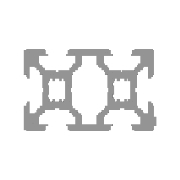
# Autodesk Inventor part: 2040Vslot
Saved by Autodesk Inventor 2023 (Build 270158000, 158)
## iProperties
IsCustomPart: 1
Created: 2023-08-15
Part Number: 2040Vslot
Material: Aluminum 6061
Description: STEP AP214
Document SubType Name: Modeling
Designer: Felix
Language: en-US
Size Designation: (Unnamed 1)
Categories: <MemberInstance><Categories><Category DisplayName="Structural Shapes" InternalName="089c4875-fa83-4c05-b084-43b9cc11f5ed" Mnemonic="GRDR"><CategoryParameter DisplayName="Mass per Length Unit" InternalName="0bb95a10-148f-4027-a459-38d7b056702a" Mnemonic="shpmass"/><CategoryParameter DisplayName="Section Area" InternalName="1ff91680-64b0-4202-b9a3-7fd3f94bba3b" Mnemonic="secarea"/><CategoryParameter DisplayName="Radius of Gyration (x)" InternalName="25778675-03e9-40c1-b6a8-4a9ed693320d" Mnemonic="gyrradx"/><CategoryParameter DisplayName="Torsional Rigidity Modulus" InternalName="26c1ec35-5026-4c63-ad0a-751cf684a536" Mnemonic="torrigmod"/><CategoryParameter DisplayName="Distance of the Center of Gravity X-X" InternalName="26c9bdb8-9c79-4b4f-a92e-8e197583c9c4" Mnemonic="grcendistX"/><CategoryParameter DisplayName="Legacy Member ID" InternalName="340afe4f-75d7-48d3-ab7d-943f3c3da468" Mnemonic="LegacyMemberID"/><CategoryParameter DisplayName="Base Length" InternalName="42e34263-8f20-4d0e-ad48-bf1385b87c24" Mnemonic="shplen"/><CategoryParameter DisplayName="Moment of Inertia (y)" InternalName="4b9f58ea-bced-460e-81ea-3d29ca5a49e3" Mnemonic="inermomy"/><CategoryParameter DisplayName="Moment of Inertia (x)" InternalName="4cd780bc-73d7-43ac-917a-579e5cbd684d" Mnemonic="inermomx"/><CategoryParameter DisplayName="Custom Base Point" InternalName="4f1d1b73-316d-484b-a3df-9cbabb16eb77" Mnemonic="shpBasePoint"/><CategoryParameter DisplayName="Shape Height" InternalName="50274e7d-5ac0-4796-92cb-c59e54983c67" Mnemonic="shpheig"/><CategoryParameter DisplayName="Section Module (y)" InternalName="59eaa5e9-d227-48dc-b6c1-6920f96e0f95" Mnemonic="secmody"/><CategoryParameter DisplayName="Section Designation" InternalName="5a64d034-428d-49c8-ba32-7619764de20f" Mnemonic="shpdes"/><CategoryParameter DisplayName="Section Module (x)" InternalName="72cfad18-cf51-4ed4-aaa7-c6b224f8419f" Mnemonic="secmodx"/><CategoryParameter DisplayName="Torsional Section Modulus" InternalName="7c55a8dc-8844-49f9-a867-cc677b30ec9a" Mnemonic="torsecmod"/><CategoryParameter DisplayName="Shape Width" InternalName="7c717d54-a18f-4666-b4d4-573cce22c62c" Mnemonic="shpwdth"/><CategoryParameter DisplayName="Second Shape Thickness" InternalName="9251a8e1-85fd-4e47-af99-afdb762317d9" Mnemonic="shpthick2"/><CategoryParameter DisplayName="FG Authored" InternalName="9c666724-f362-4ea7-ac62-f6a007de5c69" Mnemonic="shpFGAuto"/><CategoryParameter DisplayName="Distance of the Center of Gravity Y-Y" InternalName="bcc4fb17-7af4-436a-8f8c-d0aa3b0248c5" Mnemonic="grcendistY"/><CategoryParameter DisplayName="Radius of Gyration (y)" InternalName="bfa18ebe-1636-4dbe-8d42-b263e0b73184" Mnemonic="gyrrady"/><CategoryParameter DisplayName="Shape Thickness" InternalName="d109cf76-8eb4-42fc-9800-4409734adc67" Mnemonic="shpthick"/><CategoryParameter DisplayName="Coefficient of Shear Displacement" InternalName="de4c90c6-aaa8-468f-a335-6737b311b5d3" Mnemonic="shdispc"/><Category DisplayName="Other" InternalName="f02205ff-2390-476f-921c-0b3185f88e84" Mnemonic="OTHSHP"><CategoryParameter DisplayName="Moment of Inertia (y)" InternalName="044c654e-f649-48ac-84cc-650a29ae31ca" Mnemonic="inermomy"/><CategoryParameter DisplayName="Shape Thickness" InternalName="12b1a788-9233-48fd-a933-2df8ff42b15f" Mnemonic="shpthick"/><CategoryParameter DisplayName="Mass per Length Unit" InternalName="2fd289d6-9394-4d2d-97e6-6659d7d4551d" Mnemonic="shpmass"/><CategoryParameter DisplayName="Radius of Gyration (y)" InternalName="743e1dfe-1bba-408b-b985-cf752b207386" Mnemonic="gyrrady"/><CategoryParameter DisplayName="Section Module (y)" InternalName="88b8bff9-a616-4028-93d5-ed4f79680d13" Mnemonic="secmody"/><CategoryParameter DisplayName="Section Area" InternalName="c46ecdf8-b6eb-4db9-8b25-30258930c1e3" Mnemonic="secarea"/><CategoryParameter DisplayName="Section Module (x)" InternalName="cac70804-9d39-43bb-be17-56ea1f39a6c2" Mnemonic="secmodx"/><CategoryParameter DisplayName="Moment of Inertia (x)" InternalName="ec6737bc-264f-43ed-b0bd-f6d410c2718d" Mnemonic="inermomx"/><CategoryParameter DisplayName="Radius of Gyration (x)" InternalName="ee72c61e-565e-4fd6-b448-66e1e1abcb7e" Mnemonic="gyrradx"/></Category></Category><Category DisplayName="DataType" InternalName="23b78d0f-2648-40c6-8793-ca6db495c9e8" Mnemonic="DATATYPE"><CategoryParameter DisplayName="DisplayName" InternalName="05415f3d-3907-474b-a020-eb9d644f4cf3" Mnemonic="DISPLAYNAME"/><CategoryParameter DisplayName="Standard" InternalName="0c0a119c-1e12-4c84-803f-101930972f5e" Mnemonic="STANDARD"/><CategoryParameter DisplayName="Description" InternalName="13903e3d-64b1-4950-80da-f627842ea37f" Mnemonic="DESCRIPTION"/><CategoryParameter DisplayName="Designation" InternalName="2675968c-4ce5-49e0-a4f5-552d29089031" Mnemonic="DESIGNATION"/><CategoryParameter DisplayName="Default Row" InternalName="2af9ec52-faaa-4026-b378-f9fa4afca842" Mnemonic="DEFAULTROW"/><CategoryParameter DisplayName="Folder Name" InternalName="3f06958e-8713-4116-9be7-ed6184ecc97b" Mnemonic="FOLDERNAME"/><CategoryParameter DisplayName="Revision Guid" InternalName="45a75005-10b1-4dfc-8d6d-dfe629f0b93c" Mnemonic="REVISIONGUID"/><CategoryParameter DisplayName="FileName" InternalName="8b46a4cc-9585-4fed-90c3-899f57e09a73" Mnemonic="FILENAME"/><CategoryParameter DisplayName="StdsOrg" InternalName="8f5914e1-4693-403f-8ab5-d37768198c9d" Mnemonic="STDSORG"/><CategoryParameter DisplayName="Family Version" InternalName="914462f6-6e19-4b14-ba84-155b9680b1d0" Mnemonic="FAMILYREVISION"/><CategoryParameter DisplayName="Standard Revision" InternalName="91d5a463-65c2-4fde-b823-3b7fea5e8e17" Mnemonic="STANDARDREVISION"/><CategoryParameter DisplayName="Member Revision" InternalName="a65d44b9-392f-4f4f-857b-e4b3d54996fe" Mnemonic="MEMBERREVISION"/><CategoryParameter DisplayName="ClipFormat" InternalName="bc51e27b-3422-4e78-93ef-cec197ddf230" Mnemonic="CLIPFORMAT"/><CategoryParameter DisplayName="Manufacturer" InternalName="cd6c7a72-a28a-4e50-99a9-2c7f4e13e5ad" Mnemonic="MANUFACTURER"/><CategoryParameter DisplayName="InternalName" InternalName="cf1d0246-76d9-4b4a-8305-fa0409afb5c1" Mnemonic="INTERNALNAME"/><CategoryParameter DisplayName="IsMetric" InternalName="e2385c5b-1ea4-4823-96a8-8de651266ec3" Mnemonic="ISMETRIC"/><Category DisplayName="Part" InternalName="c0e0b642-3bcb-4cc8-9e80-f96d35c4afa4" Mnemonic="PART"><CategoryParameter DisplayName="Part Number" InternalName="016b6077-bfbe-49bd-92c9-d8d59c39c941" Mnemonic="PARTNUMBER"/><CategoryParameter DisplayName="Stock Number" InternalName="4dba7c1c-e26c-444e-836c-b08b433409a8" Mnemonic="STOCKNUMBER"/><CategoryParameter DisplayName="Material Key" InternalName="5c9a8adb-dd2b-4535-b97f-0a94a95fe41f" Mnemonic="MATERIALKEY"/><CategoryParameter DisplayName="Material" InternalName="818a152a-d3c3-49ca-80ee-df7d91421b8e" Mnemonic="MATERIAL"/></Category></Category></Categories><FamilyTemplate Id="2040Vslot"><FamilyTemplateParameters><FamilyTemplateParameter ObjectType="kUserParameterObject" ValueType="xs:double" Id="12" ObjectReferenceKey="LENGTH"/><FamilyTemplateParameter ObjectType="kPartComponentDefinitionObject" ValueType="xs:string" Id="23" SubObjectId="Material"/><FamilyTemplateParameter ObjectType="kPropertyObject" ValueType="xs:string" Id="26" ObjectReferenceKey="{32853F0F-3444-11d1-9E93-0060B03C1CA6}" SubObjectId="5"/><FamilyTemplateParameter ObjectType="kPropertyObject" ValueType="xs:string" Id="27" ObjectReferenceKey="{32853F0F-3444-11d1-9E93-0060B03C1CA6}" SubObjectId="52"/></FamilyTemplateParameters></FamilyTemplate><CategoryParameterMap><ParamToTemplateMap><ParamToTemplate CategoryParameter="//CategoryParameter[@InternalName='cf1d0246-76d9-4b4a-8305-fa0409afb5c1']" ConstantValue="7aca6009-b639-4b80-b43f-4fabf888ce7f"/><ParamToTemplate CategoryParameter="//CategoryParameter[@InternalName='45a75005-10b1-4dfc-8d6d-dfe629f0b93c']" ConstantValue="1da94dc8-9529-43b5-a307-749102fad576"/><ParamToTemplate CategoryParameter="//CategoryParameter[@InternalName='3f06958e-8713-4116-9be7-ed6184ecc97b']" ConstantValue="2040Vslot"/><ParamToTemplate CategoryParameter="//CategoryParameter[@InternalName='8f5914e1-4693-403f-8ab5-d37768198c9d']" TemplateParameter="17"/><ParamToTemplate CategoryParameter="//CategoryParameter[@InternalName='0c0a119c-1e12-4c84-803f-101930972f5e']" TemplateParameter="18"/><ParamToTemplate CategoryParameter="//CategoryParameter[@InternalName='91d5a463-65c2-4fde-b823-3b7fea5e8e17']" TemplateParameter="19"/><ParamToTemplate CategoryParameter="//CategoryParameter[@InternalName='cd6c7a72-a28a-4e50-99a9-2c7f4e13e5ad']" TemplateParameter="20"/><ParamToTemplate CategoryParameter="//CategoryParameter[@InternalName='13903e3d-64b1-4950-80da-f627842ea37f']" ConstantValue="STEP AP214"/><ParamToTemplate CategoryParameter="//CategoryParameter[@InternalName='05415f3d-3907-474b-a020-eb9d644f4cf3']" ConstantValue="2040Vslot"/><ParamToTemplate CategoryParameter="//CategoryParameter[@InternalName='914462f6-6e19-4b14-ba84-155b9680b1d0']" ConstantValue="11"/><ParamToTemplate CategoryParameter="//CategoryParameter[@InternalName='bc51e27b-3422-4e78-93ef-cec197ddf230']" ConstantValue="CF_INVENTOR.STDPARTS"/><ParamToTemplate CategoryParameter="//CategoryParameter[@InternalName='e2385c5b-1ea4-4823-96a8-8de651266ec3']" ConstantValue="true"/><ParamToTemplate CategoryParameter="//CategoryParameter[@InternalName='2af9ec52-faaa-4026-b378-f9fa4afca842']" ConstantValue="1"/><ParamToTemplate CategoryParameter="//CategoryParameter[@InternalName='9c666724-f362-4ea7-ac62-f6a007de5c69']" ConstantValue="1"/><ParamToTemplate CategoryParameter="//CategoryParameter[@InternalName='8b46a4cc-9585-4fed-90c3-899f57e09a73']" ConstantValue="1"/><ParamToTemplate CategoryParameter="//CategoryParameter[@InternalName='a65d44b9-392f-4f4f-857b-e4b3d54996fe']" ConstantValue="3427034b-88d6-4288-aace-d63c815935a5"/><ParamToTemplate CategoryParameter="//CategoryParameter[@InternalName='a65d44b9-392f-4f4f-857b-e4b3d54996fe']" ConstantValue="3427034b-88d6-4288-aace-d63c815935a5"/><ParamToTemplate CategoryParameter="//CategoryParameter[@InternalName='2675968c-4ce5-49e0-a4f5-552d29089031']" TemplateParameter="27"/><ParamToTemplate CategoryParameter="//CategoryParameter[@InternalName='42e34263-8f20-4d0e-ad48-bf1385b87c24']" TemplateParameter="12"/><ParamToTemplate CategoryParameter="//CategoryParameter[@InternalName='818a152a-d3c3-49ca-80ee-df7d91421b8e']" TemplateParameter="23"/><ParamToTemplate CategoryParameter="//CategoryParameter[@InternalName='016b6077-bfbe-49bd-92c9-d8d59c39c941']" TemplateParameter="26"/></ParamToTemplateMap></CategoryParameterMap></MemberInstance>
Density: 2.7 g/cm^3
Appearance: Aluminum - Flat
_CCFamilyDisplayName: 2040Vslot - STEP AP214
_FrameMemberDoc: Frame Member File
_Version: 25.0.0
_GetPNFromCC: 1
Sending System: SolidWorks 2018
Preprocessor: SwSTEP 2.0
G_L: 730,000 mm
G_W: 40,000 mm
G_H: 20,000 mm
+5D53ACFD-2916-4EAC-BA86-D05F515BD30D+CUTDETAIL1: Length Change
Title: 2040x100 Vslot.STEP
Author: Felix
Autodesk Inventor part; units mm, degrees
ref_plane "YZ Plane" through (0, 0, 0) normal (1, 0, 0) x (0, 1, 0)
ref_plane "XZ Plane" through (0, 0, 0) normal (0, 1, 0) x (-1, 0, 0)
ref_plane "XY Plane" through (0, 0, 0) normal (0, 0, 1) x (1, 0, 0)
ref_plane "Work Plane3" through (0.5, 0, 50) normal (0, 0, 1) x (1, 0, 0)
ref_plane "Start Plane" through (0.5, 0, 10) normal (0, 0, 1) x (1, 0, 0)
ref_plane "End Plane" through (0.5, 0, 740) normal (0, 0, 1) x (1, 0, 0)
sketch "Sketch" plane through (0.5, 0, 50) normal (0, 0, 1) x (1, 0, 0)
  arc A0 (-12.7, 20) -> (-14.2, 18.5) centre (-12.7, 18.5) ccw projected
  line L0 (-14.2, 18.5) -> (-14.2, 14.2) projected
  line L1 (-14.2, 14.2) -> (-13, 13) projected
  line L2 (-13, 13) -> (-12.7, 13) projected
  line L3 (-12.7, 13) -> (-12.7, 15.5) projected
  arc A1 (-12.2, 16) -> (-12.7, 15.5) centre (-12.2, 15.5) ccw projected
  line L4 (-12.2, 16) -> (-11.4678, 16) projected
  arc A2 (-11.1142, 15.8536) -> (-11.4678, 16) centre (-11.4678, 15.5) ccw projected
  line L5 (-11.1142, 15.8536) -> (-8.8464, 13.5858) projected
  arc A3 (-8.7, 13.2322) -> (-8.8464, 13.5858) centre (-9.2, 13.2322) ccw projected
  line L6 (-8.7, 13.2322) -> (-8.7, 10.9536) projected
  arc A4 (-8.7, 10.9536) -> (-8.6732, 10.8536) centre (-8.5, 10.9536) ccw projected
  line L7 (-8.6732, 10.8536) -> (-8.2381, 10.1) projected
  arc A5 (-8.2381, 9.9) -> (-8.2381, 10.1) centre (-8.4113, 10) ccw projected
  line L8 (-8.2381, 9.9) -> (-8.6732, 9.1464) projected
  arc A6 (-8.6732, 9.1464) -> (-8.7, 9.0464) centre (-8.5, 9.0464) ccw projected
  line L9 (-8.7, 9.0464) -> (-8.7, 6.7678) projected
  arc A7 (-8.8464, 6.4142) -> (-8.7, 6.7678) centre (-9.2, 6.7678) ccw projected
  line L10 (-8.8464, 6.4142) -> (-11.1142, 4.1464) projected
  arc A8 (-11.4678, 4) -> (-11.1142, 4.1464) centre (-11.4678, 4.5) ccw projected
  line L11 (-11.4678, 4) -> (-12.2, 4) projected
  arc A9 (-12.7, 4.5) -> (-12.2, 4) centre (-12.2, 4.5) ccw projected
  line L12 (-12.7, 4.5) -> (-12.7, 7) projected
  line L13 (-12.7, 7) -> (-13, 7) projected
  line L14 (-13, 7) -> (-14.2, 5.8) projected
  line L15 (-14.2, 5.8) -> (-14.2, 1.5) projected
  arc A10 (-14.2, 1.5) -> (-12.7, 0) centre (-12.7, 1.5) ccw projected
  line L16 (-12.7, 0) -> (-8.4, 0) projected
  line L17 (-8.4, 0) -> (-7.2, 1.2) projected
  line L18 (-7.2, 1.2) -> (-7.2, 1.5) projected
  line L19 (-7.2, 1.5) -> (-9.7, 1.5) projected
  arc A11 (-10.2, 2) -> (-9.7, 1.5) centre (-9.7, 2) ccw projected
  line L20 (-10.2, 2) -> (-10.2, 2.7322) projected
  arc A12 (-10.0536, 3.0858) -> (-10.2, 2.7322) centre (-9.7, 2.7322) ccw projected
  line L21 (-10.0536, 3.0858) -> (-7.7858, 5.3536) projected
  arc A13 (-7.4322, 5.5) -> (-7.7858, 5.3536) centre (-7.4322, 5) ccw projected
  line L22 (-7.4322, 5.5) -> (-5.1536, 5.5) projected
  arc A14 (-5.1536, 5.5) -> (-5.0536, 5.5268) centre (-5.1536, 5.7) ccw projected
  line L23 (-5.0536, 5.5268) -> (-4.3, 5.9619) projected
  arc A15 (-4.1, 5.9619) -> (-4.3, 5.9619) centre (-4.2, 5.7887) ccw projected
  line L24 (-4.1, 5.9619) -> (-3.3464, 5.5268) projected
  arc A16 (-3.3464, 5.5268) -> (-3.2464, 5.5) centre (-3.2464, 5.7) ccw projected
  line L25 (-3.2464, 5.5) -> (-0.9678, 5.5) projected
  arc A17 (-0.6142, 5.3536) -> (-0.9678, 5.5) centre (-0.9678, 5) ccw projected
  line L26 (-0.6142, 5.3536) -> (1.6536, 3.0858) projected
  arc A18 (1.8, 2.7322) -> (1.6536, 3.0858) centre (1.3, 2.7322) ccw projected
  line L27 (1.8, 2.7322) -> (1.8, 2) projected
  arc A19 (1.3, 1.5) -> (1.8, 2) centre (1.3, 2) ccw projected
  line L28 (1.3, 1.5) -> (-1.2, 1.5) projected
  line L29 (-1.2, 1.5) -> (-1.2, 1.2) projected
  line L30 (-1.2, 1.2) -> (0, 0) projected
  line L31 (0, 0) -> (11.6, 0) projected
  line L32 (11.6, 0) -> (12.8, 1.2) projected
  line L33 (12.8, 1.2) -> (12.8, 1.5) projected
  line L34 (12.8, 1.5) -> (10.3, 1.5) projected
  arc A20 (9.8, 2) -> (10.3, 1.5) centre (10.3, 2) ccw projected
  line L35 (9.8, 2) -> (9.8, 2.7322) projected
  arc A21 (9.9464, 3.0858) -> (9.8, 2.7322) centre (10.3, 2.7322) ccw projected
  line L36 (9.9464, 3.0858) -> (12.2142, 5.3536) projected
  arc A22 (12.5678, 5.5) -> (12.2142, 5.3536) centre (12.5678, 5) ccw projected
  line L37 (12.5678, 5.5) -> (14.8464, 5.5) projected
  arc A23 (14.8464, 5.5) -> (14.9464, 5.5268) centre (14.8464, 5.7) ccw projected
  line L38 (14.9464, 5.5268) -> (15.7, 5.9619) projected
  arc A24 (15.9, 5.9619) -> (15.7, 5.9619) centre (15.8, 5.7887) ccw projected
  line L39 (15.9, 5.9619) -> (16.6536, 5.5268) projected
  arc A25 (16.6536, 5.5268) -> (16.7536, 5.5) centre (16.7536, 5.7) ccw projected
  line L40 (16.7536, 5.5) -> (19.0322, 5.5) projected
  arc A26 (19.3858, 5.3536) -> (19.0322, 5.5) centre (19.0322, 5) ccw projected
  line L41 (19.3858, 5.3536) -> (21.6536, 3.0858) projected
  arc A27 (21.8, 2.7322) -> (21.6536, 3.0858) centre (21.3, 2.7322) ccw projected
  line L42 (21.8, 2.7322) -> (21.8, 2) projected
  arc A28 (21.3, 1.5) -> (21.8, 2) centre (21.3, 2) ccw projected
  line L43 (21.3, 1.5) -> (18.8, 1.5) projected
  line L44 (18.8, 1.5) -> (18.8, 1.2) projected
  line L45 (18.8, 1.2) -> (20, 0) projected
  line L46 (20, 0) -> (24.3, 0) projected
  arc A29 (24.3, 0) -> (25.8, 1.5) centre (24.3, 1.5) ccw projected
  line L47 (25.8, 1.5) -> (25.8, 5.8) projected
  line L48 (25.8, 5.8) -> (24.6, 7) projected
  line L49 (24.6, 7) -> (24.3, 7) projected
  line L50 (24.3, 7) -> (24.3, 4.5) projected
  arc A30 (23.8, 4) -> (24.3, 4.5) centre (23.8, 4.5) ccw projected
  line L51 (23.8, 4) -> (23.0678, 4) projected
  arc A31 (22.7142, 4.1464) -> (23.0678, 4) centre (23.0678, 4.5) ccw projected
  line L52 (22.7142, 4.1464) -> (20.4464, 6.4142) projected
  arc A32 (20.3, 6.7678) -> (20.4464, 6.4142) centre (20.8, 6.7678) ccw projected
  line L53 (20.3, 6.7678) -> (20.3, 9.0464) projected
  arc A33 (20.3, 9.0464) -> (20.2732, 9.1464) centre (20.1, 9.0464) ccw projected
  line L54 (20.2732, 9.1464) -> (19.8381, 9.9) projected
  arc A34 (19.8381, 10.1) -> (19.8381, 9.9) centre (20.0113, 10) ccw projected
  line L55 (19.8381, 10.1) -> (20.2732, 10.8536) projected
  arc A35 (20.2732, 10.8536) -> (20.3, 10.9536) centre (20.1, 10.9536) ccw projected
  line L56 (20.3, 10.9536) -> (20.3, 13.2322) projected
  arc A36 (20.4464, 13.5858) -> (20.3, 13.2322) centre (20.8, 13.2322) ccw projected
  line L57 (20.4464, 13.5858) -> (22.7142, 15.8536) projected
  arc A37 (23.0678, 16) -> (22.7142, 15.8536) centre (23.0678, 15.5) ccw projected
  line L58 (23.0678, 16) -> (23.8, 16) projected
  arc A38 (24.3, 15.5) -> (23.8, 16) centre (23.8, 15.5) ccw projected
  line L59 (24.3, 15.5) -> (24.3, 13) projected
  line L60 (24.3, 13) -> (24.6, 13) projected
  line L61 (24.6, 13) -> (25.8, 14.2) projected
  line L62 (25.8, 14.2) -> (25.8, 18.5) projected
  arc A39 (25.8, 18.5) -> (24.3, 20) centre (24.3, 18.5) ccw projected
  line L63 (24.3, 20) -> (20, 20) projected
  line L64 (20, 20) -> (18.8, 18.8) projected
  line L65 (18.8, 18.8) -> (18.8, 18.5) projected
  line L66 (18.8, 18.5) -> (21.3, 18.5) projected
  arc A40 (21.8, 18) -> (21.3, 18.5) centre (21.3, 18) ccw projected
  line L67 (21.8, 18) -> (21.8, 17.2678) projected
  arc A41 (21.6536, 16.9142) -> (21.8, 17.2678) centre (21.3, 17.2678) ccw projected
  line L68 (21.6536, 16.9142) -> (19.3858, 14.6464) projected
  arc A42 (19.0322, 14.5) -> (19.3858, 14.6464) centre (19.0322, 15) ccw projected
  line L69 (19.0322, 14.5) -> (16.7536, 14.5) projected
  arc A43 (16.7536, 14.5) -> (16.6536, 14.4732) centre (16.7536, 14.3) ccw projected
  line L70 (16.6536, 14.4732) -> (15.9, 14.0381) projected
  arc A44 (15.7, 14.0381) -> (15.9, 14.0381) centre (15.8, 14.2113) ccw projected
  line L71 (15.7, 14.0381) -> (14.9464, 14.4732) projected
  arc A45 (14.9464, 14.4732) -> (14.8464, 14.5) centre (14.8464, 14.3) ccw projected
  line L72 (14.8464, 14.5) -> (12.5678, 14.5) projected
  arc A46 (12.2142, 14.6464) -> (12.5678, 14.5) centre (12.5678, 15) ccw projected
  line L73 (12.2142, 14.6464) -> (9.9464, 16.9142) projected
  arc A47 (9.8, 17.2678) -> (9.9464, 16.9142) centre (10.3, 17.2678) ccw projected
  line L74 (9.8, 17.2678) -> (9.8, 18) projected
  arc A48 (10.3, 18.5) -> (9.8, 18) centre (10.3, 18) ccw projected
  line L75 (10.3, 18.5) -> (12.8, 18.5) projected
  line L76 (12.8, 18.5) -> (12.8, 18.8) projected
  line L77 (12.8, 18.8) -> (11.6, 20) projected
  line L78 (11.6, 20) -> (0, 20) projected
  line L79 (0, 20) -> (-1.2, 18.8) projected
  line L80 (-1.2, 18.8) -> (-1.2, 18.5) projected
  line L81 (-1.2, 18.5) -> (1.3, 18.5) projected
  arc A49 (1.8, 18) -> (1.3, 18.5) centre (1.3, 18) ccw projected
  line L82 (1.8, 18) -> (1.8, 17.2678) projected
  arc A50 (1.6536, 16.9142) -> (1.8, 17.2678) centre (1.3, 17.2678) ccw projected
  line L83 (1.6536, 16.9142) -> (-0.6142, 14.6464) projected
  arc A51 (-0.9678, 14.5) -> (-0.6142, 14.6464) centre (-0.9678, 15) ccw projected
  line L84 (-0.9678, 14.5) -> (-3.2464, 14.5) projected
  arc A52 (-3.2464, 14.5) -> (-3.3464, 14.4732) centre (-3.2464, 14.3) ccw projected
  line L85 (-3.3464, 14.4732) -> (-4.1, 14.0381) projected
  arc A53 (-4.3, 14.0381) -> (-4.1, 14.0381) centre (-4.2, 14.2113) ccw projected
  line L86 (-4.3, 14.0381) -> (-5.0536, 14.4732) projected
  arc A54 (-5.0536, 14.4732) -> (-5.1536, 14.5) centre (-5.1536, 14.3) ccw projected
  line L87 (-5.1536, 14.5) -> (-7.4322, 14.5) projected
  arc A55 (-7.7858, 14.6464) -> (-7.4322, 14.5) centre (-7.4322, 15) ccw projected
  line L88 (-7.7858, 14.6464) -> (-10.0536, 16.9142) projected
  arc A56 (-10.2, 17.2678) -> (-10.0536, 16.9142) centre (-9.7, 17.2678) ccw projected
  line L89 (-10.2, 17.2678) -> (-10.2, 18) projected
  arc A57 (-9.7, 18.5) -> (-10.2, 18) centre (-9.7, 18) ccw projected
  line L90 (-9.7, 18.5) -> (-7.2, 18.5) projected
  line L91 (-7.2, 18.5) -> (-7.2, 18.8) projected
  line L92 (-7.2, 18.8) -> (-8.4, 20) projected
  line L93 (-8.4, 20) -> (-12.7, 20) projected
  line L94 (17.0582, 7.5547) -> (17.7099, 7.0078) projected
  arc A58 (14.5418, 7.5547) -> (17.0582, 7.5547) centre (15.8, 10) ccw projected
  line L95 (13.8901, 7.0078) -> (14.5418, 7.5547) projected
  arc A59 (12.8104, 8.0861) -> (13.8901, 7.0078) centre (15.8, 10) ccw projected
  line L96 (13.3547, 8.7418) -> (12.8104, 8.0861) projected
  arc A60 (13.3547, 11.2582) -> (13.3547, 8.7418) centre (15.8, 10) ccw projected
  line L97 (12.8104, 11.9139) -> (13.3547, 11.2582) projected
  arc A61 (13.8901, 12.9922) -> (12.8104, 11.9139) centre (15.8, 10) ccw projected
  line L98 (14.5418, 12.4453) -> (13.8901, 12.9922) projected
  arc A62 (17.0582, 12.4453) -> (14.5418, 12.4453) centre (15.8, 10) ccw projected
  line L99 (17.7099, 12.9922) -> (17.0582, 12.4453) projected
  arc A63 (18.7896, 11.9139) -> (17.7099, 12.9922) centre (15.8, 10) ccw projected
  line L100 (18.2453, 11.2582) -> (18.7896, 11.9139) projected
  arc A64 (18.2453, 8.7418) -> (18.2453, 11.2582) centre (15.8, 10) ccw projected
  line L101 (18.7896, 8.0861) -> (18.2453, 8.7418) projected
  arc A65 (17.7099, 7.0078) -> (18.7896, 8.0861) centre (15.8, 10) ccw projected
  line L102 (-2.9418, 7.5547) -> (-2.2901, 7.0078) projected
  arc A66 (-5.4582, 7.5547) -> (-2.9418, 7.5547) centre (-4.2, 10) ccw projected
  line L103 (-6.1099, 7.0078) -> (-5.4582, 7.5547) projected
  arc A67 (-7.1896, 8.0861) -> (-6.1099, 7.0078) centre (-4.2, 10) ccw projected
  line L104 (-6.6453, 8.7418) -> (-7.1896, 8.0861) projected
  arc A68 (-6.6453, 11.2582) -> (-6.6453, 8.7418) centre (-4.2, 10) ccw projected
  line L105 (-7.1896, 11.9139) -> (-6.6453, 11.2582) projected
  arc A69 (-6.1099, 12.9922) -> (-7.1896, 11.9139) centre (-4.2, 10) ccw projected
  line L106 (-5.4582, 12.4453) -> (-6.1099, 12.9922) projected
  arc A70 (-2.9418, 12.4453) -> (-5.4582, 12.4453) centre (-4.2, 10) ccw projected
  line L107 (-2.2901, 12.9922) -> (-2.9418, 12.4453) projected
  arc A71 (-1.2104, 11.9139) -> (-2.2901, 12.9922) centre (-4.2, 10) ccw projected
  line L108 (-1.7547, 11.2582) -> (-1.2104, 11.9139) projected
  arc A72 (-1.7547, 8.7418) -> (-1.7547, 11.2582) centre (-4.2, 10) ccw projected
  line L109 (-1.2104, 8.0861) -> (-1.7547, 8.7418) projected
  arc A73 (-2.2901, 7.0078) -> (-1.2104, 8.0861) centre (-4.2, 10) ccw projected
  line L110 (3.8, 1.5) -> (7.8, 1.5) projected
  arc A74 (3.3, 2) -> (3.8, 1.5) centre (3.8, 2) ccw projected
  line L111 (3.3, 3.3536) -> (3.3, 2) projected
  arc A75 (3.3, 3.3536) -> (3.1536, 3.7071) centre (2.8, 3.3536) ccw projected
  line L112 (0.4464, 6.4142) -> (3.1536, 3.7071) projected
  arc A76 (0.3, 6.7678) -> (0.4464, 6.4142) centre (0.8, 6.7678) ccw projected
  line L113 (0.3, 9.0464) -> (0.3, 6.7678) projected
  arc A77 (0.3, 9.0464) -> (0.2732, 9.1464) centre (0.1, 9.0464) ccw projected
  line L114 (-0.1619, 9.9) -> (0.2732, 9.1464) projected
  arc A78 (-0.1619, 10.1) -> (-0.1619, 9.9) centre (0.0113, 10) ccw projected
  line L115 (0.2732, 10.8536) -> (-0.1619, 10.1) projected
  arc A79 (0.2732, 10.8536) -> (0.3, 10.9536) centre (0.1, 10.9536) ccw projected
  line L116 (0.3, 13.2322) -> (0.3, 10.9536) projected
  arc A80 (0.4464, 13.5858) -> (0.3, 13.2322) centre (0.8, 13.2322) ccw projected
  line L117 (3.1536, 16.2929) -> (0.4464, 13.5858) projected
  arc A81 (3.1536, 16.2929) -> (3.3, 16.6464) centre (2.8, 16.6464) ccw projected
  line L118 (3.3, 18) -> (3.3, 16.6464) projected
  arc A82 (3.8, 18.5) -> (3.3, 18) centre (3.8, 18) ccw projected
  line L119 (7.8, 18.5) -> (3.8, 18.5) projected
  arc A83 (8.3, 18) -> (7.8, 18.5) centre (7.8, 18) ccw projected
  line L120 (8.3, 16.6464) -> (8.3, 18) projected
  arc A84 (8.3, 16.6464) -> (8.4464, 16.2929) centre (8.8, 16.6464) ccw projected
  line L121 (11.1536, 13.5858) -> (8.4464, 16.2929) projected
  arc A85 (11.3, 13.2322) -> (11.1536, 13.5858) centre (10.8, 13.2322) ccw projected
  line L122 (11.3, 10.9536) -> (11.3, 13.2322) projected
  arc A86 (11.3, 10.9536) -> (11.3268, 10.8536) centre (11.5, 10.9536) ccw projected
  line L123 (11.7619, 10.1) -> (11.3268, 10.8536) projected
  arc A87 (11.7619, 9.9) -> (11.7619, 10.1) centre (11.5887, 10) ccw projected
  line L124 (11.3268, 9.1464) -> (11.7619, 9.9) projected
  arc A88 (11.3268, 9.1464) -> (11.3, 9.0464) centre (11.5, 9.0464) ccw projected
  line L125 (11.3, 6.7678) -> (11.3, 9.0464) projected
  arc A89 (11.1536, 6.4142) -> (11.3, 6.7678) centre (10.8, 6.7678) ccw projected
  line L126 (8.4464, 3.7071) -> (11.1536, 6.4142) projected
  arc A90 (8.4464, 3.7071) -> (8.3, 3.3536) centre (8.8, 3.3536) ccw projected
  line L127 (8.3, 2) -> (8.3, 3.3536) projected
  arc A91 (7.8, 1.5) -> (8.3, 2) centre (7.8, 2) ccw projected
  point P0 (-0.5, 0)
extrude "Body" add sketch "Sketch" along normal up to surface (730 mm away) from surface at -40
sketch "Sketch4" plane through (0.5, 0, 50) normal (0, 0, 1) x (1, 0, 0)
  line L0 (0, 0) -> (10, 0)
ref_plane "Work Plane7" through (0.5, 0, 50) normal (0, -1, 0) x (1, 0, 0)
sketch "Sketch5" plane through (0.5, 0, 50) normal (0, -1, 0) x (1, 0, 0)
  line L0 (-2, -40) -> (12, -40)
  line L1 (-2, 690) -> (12, 690)
  dimension "d7" = 730
  measures "d7" distance between parallel lines of L0 L1
equation "\"G_L\" = d7"
body "Solid2"
